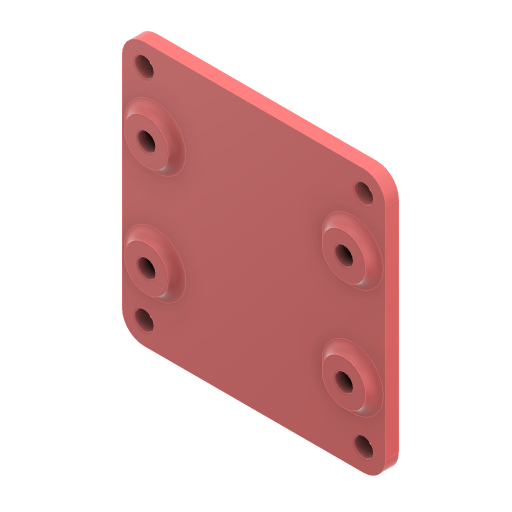
# Autodesk Inventor part: power_distribution_mount
Saved by Autodesk Inventor 2023 (Build 270158000, 158)
## iProperties
Created: 2024-05-10
Part Number: power_distribution_mount
Material: Generic
Document SubType Name: Modeling
Designer: Thomas
Density: 1 g/cm^3
Appearance: Smooth - Red
Author: Thomas
Autodesk Inventor part; units mm, degrees
ref_plane "YZ Plane" through (0, 0, 0) normal (1, 0, 0) x (0, 1, 0)
ref_plane "XZ Plane" through (0, 0, 0) normal (0, 1, 0) x (-1, 0, 0)
ref_plane "XY Plane" through (0, 0, 0) normal (0, 0, 1) x (1, 0, 0)
sketch "Sketch1" plane through (0, 0, 0) normal (0, 0, 1) x (1, 0, 0)
  line L0 (0, 0) -> (60, 0)
  line L1 (60, 0) -> (60, 60)
  line L2 (60, 60) -> (0, 60)
  line L3 (0, 60) -> (0, 0)
  line L4 (5, 55) -> (55, 55) construction
  line L5 (55, 55) -> (55, 5) construction
  line L6 (55, 5) -> (5, 5) construction
  line L7 (5, 5) -> (5, 55) construction
  circle A0 centre (5, 55) radius 2.2
  circle A1 centre (55, 55) radius 2.2
  circle A2 centre (55, 5) radius 2.2
  circle A3 centre (5, 5) radius 2.2
  line L8 (7.5, 42.5) -> (52.5, 42.5) construction
  line L9 (52.5, 42.5) -> (52.5, 17.5) construction
  line L10 (52.5, 17.5) -> (7.5, 17.5) construction
  line L11 (7.5, 17.5) -> (7.5, 42.5) construction
  circle A4 centre (7.5, 42.5) radius 5
  circle A5 centre (7.5, 42.5) radius 2.1
  dimension "d0" = 60
  dimension "d1" = 60
  dimension "d2" = 50
  dimension "d3" = 50
  dimension "d4" = 5
  dimension "d5" = 5
  dimension "d6" = 4.4
  dimension "d7" = 4.4
  dimension "d8" = 4.4
  dimension "d9" = 4.4
  dimension "d10" = 45
  dimension "d11" = 25
  dimension "d12" = 17.5
  dimension "d13" = 7.5
  dimension "d14" = 10
  dimension "d15" = 4.2
  constraints: 24 end point, 10 coincident, 6 centre point, 6 parallel, 3 horizontal, 3 perpendicular
  measures "d0" distance of L2.end L1.end
  measures "d1" distance of L1.end L0.end
  measures "d2" distance of L5.end L6.end
  measures "d3" distance of L4.end L5.end
  measures "d4" distance between parallel lines of L3 L7
  measures "d5" distance between parallel lines of L2 L4
  measures "d6" diameter of A0
  measures "d7" diameter of A1
  measures "d8" diameter of A2
  measures "d9" diameter of A3
  measures "d10" distance of L9.end L10.end
  measures "d11" distance of L8.end L9.end
  measures "d12" distance between parallel lines of L8 L2
  measures "d13" distance between parallel lines of L3 L11
  measures "d14" diameter of A4
  measures "d15" diameter of A5
extrude "Extrusion1" add sketch "Sketch1" against normal blind 3 contours L3 L2 L1 L0 | A4 | A5
extrude "Extrusion2" add sketch "Sketch1" along normal blind 2 contours A4
fillet "Fillet1" radius 2 1 edges at (2.5, 42.5, 0)
extrude "Extrusion3" cut sketch "Sketch1" against normal through all contours A5
pattern_sketch "Sketch Driven Pattern1" of "Extrusion2", "Fillet1", "Extrusion3" from (7.5, 42.5, 0) copies at (52.5, 42.5, 0) at (52.5, 17.5, 0) at (7.5, 17.5, 0)
fillet "Fillet2" radius 5 4 edges at (0, 0, -1.5) (60, 0, -1.5) (60, 60, -1.5) (0, 60, -1.5)
equation "\"d4\" = -0.5 * d2 + 0.5 * d0"
equation "\"d5\" = -0.5 * d3 + 0.5 * d1"
equation "\"d12\" = -0.5 * d11 + 0.5 * d1"
equation "\"d13\" = -0.5 * d10 + 0.5 * d0"
body "Solid1"
